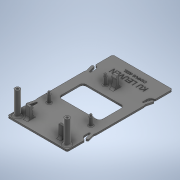
# Autodesk Inventor part: Bodemplaat_v2
Saved by Autodesk Inventor 2022 (Build 260153000, 153)
## iProperties
Created: 2022-02-17
Part Number: Bodemplaat_v2
Material: ABS Plastic
Document SubType Name: Modeling
Designer: woutr
Density: 1.06 g/cm^3
Appearance: Smooth - Black
Author: woutr
Autodesk Inventor part; units mm, degrees
note: some values were not read from the file. Chosen so that the rebuilt part matches the saved one: direction of "Emboss2".
sketch "Sketch1" plane through (0, 0, 0) normal (0, 1, 0) x (-1, 0, 0)
  line L0 (0, 0) -> (72, 0)
  line L1 (72, 0) -> (72, -127)
  line L2 (72, -127) -> (0, -127)
  line L3 (0, -127) -> (0, 0)
  line L4 (57, -50) -> (15, -50)
  line L5 (11, -54) -> (11, -76)
  line L6 (15, -80) -> (57, -80)
  line L7 (61, -76) -> (61, -54)
  arc A0 (11, -76) -> (15, -80) centre (15, -76) ccw
  arc A1 (57, -80) -> (61, -76) centre (57, -76) ccw
  arc A2 (15, -50) -> (11, -54) centre (15, -54) ccw
  arc A3 (61, -54) -> (57, -50) centre (57, -54) ccw
  point P0 (61, -50)
  point P1 (11, -80)
  point P2 (11, -50)
  point P3 (36, -50)
  point P4 (36, 0)
  dimension "d0" = 72
  dimension "d1" = 127
  dimension "d124" = 50
  dimension "d125" = 30
  dimension "d126" = 50
  dimension "d127" = 4
  constraints: 16 end point, 8 point on circle, 8 tangent, 6 point on line, 4 centre point, 4 parallel, 3 equal radius, 2 horizontal, 2 midpoint, 2 perpendicular, 1 vertical alignment
  measures "d0" distance of L1.end L2.end
  measures "d1" distance of L0.end L1.end
  measures "d124" distance between parallel lines of L0 L4
  measures "d125" distance of point (11, -50) point (11, -80)
  measures "d126" distance of point (61, -50) point (11, -50)
  measures "d127" radius of A0
extrude "Extrusion1" add sketch "Sketch1" along normal blind 2
sketch "Sketch2" plane through (0, 2, 0) normal (0, 1, 0) x (1, 0, 0)
  circle A0 centre (-60.5, 38.7) radius 2
  circle A1 centre (-11.5, 40) radius 2
  circle A2 centre (-45.2, 91.15) radius 2
  line L0 (-71, 11) -> (-1, 11) construction
  line L1 (-1, 11) -> (-1, 93.45) construction
  line L2 (-1, 93.45) -> (-71, 93.45) construction
  line L3 (-71, 93.45) -> (-71, 11) construction
  line L4 (-72, 0) -> (0, 0) projected
  point P0 (-36, 11)
  point P1 (-36, 0)
  dimension "d34" = 4
  dimension "d83" = 70
  dimension "d84" = 82.45
  dimension "d85" = 29
  dimension "d86" = 10.5
  dimension "d87" = 25.8
  dimension "d88" = 10.5
  dimension "d89" = 2.3
  dimension "d90" = 11
  dimension "d123" = 27.7
  constraints: 8 end point, 3 centre point, 2 equal radius, 2 horizontal, 2 midpoint, 2 perpendicular, 1 vertical alignment
  measures "d34" diameter of A1
  measures "d83" distance between parallel lines of L1 L3
  measures "d84" distance between parallel lines of L2 L0
  measures "d85" distance from line of L0 A1.centre
  measures "d86" distance from line of L1 A1.centre
  measures "d87" distance from line of L3 A2.centre
  measures "d88" distance from line of L3 A0.centre
  measures "d89" distance from line of L2 A2.centre
  measures "d90" distance between parallel lines of L4 L0
  measures "d123" distance from line of L0 A0.centre
extrude "Extrusion8" add sketch "Sketch2" along normal blind 9
fillet "Fillet3" radius 1 3 edges at (-62.5, 2, -38.7) (-13.5, 2, -40) (-47.2, 2, -91.15)
sketch "Sketch8" plane through (-60.5, 11, -38.7) normal (0, 1, 0) x (1, 0, 0)
  circle A0 centre (0, 0) radius 1.25
  circle A1 centre (49, 1.3) radius 2 projected
  circle A2 centre (49, 1.3) radius 1.25
  circle A3 centre (15.3, 52.45) radius 2 projected
  circle A4 centre (15.3, 52.45) radius 1.25
  circle A5 centre (0, 0) radius 2 projected
  point P0 (60.5, -38.7)
  dimension "d65" = 2.5
  dimension "d66" = 2.5
  dimension "d67" = 2.5
  constraints: 3 centre point, 2 coincident, 1 concentric
  measures "d65" diameter of A0
  measures "d66" diameter of A2
  measures "d67" diameter of A4
extrude "Extrusion9" add sketch "Sketch8" along normal blind 3 contours A0 | A2 | A4
fillet "Fillet4" radius 0.5 3 edges at (-61.75, 14, -38.7) (-12.75, 14, -40) (-46.45, 14, -91.15)
fillet "Fillet5" radius 2 4 edges at (0, 1, 0) (-72, 1, 0) (-72, 1, -127) (0, 1, -127)
ref_plane "Work Plane1" through (-16, 0, -2) normal (1, 0, 0) x (0, 0, -1)
sketch "Sketch10" plane through (-16, 0, -2) normal (1, 0, 0) x (0, 0, -1)
  line L0 (0, 2) -> (123, 2) projected
  line L1 (3.5, 2) -> (13.5, 2)
  arc A0 (10.7088, 3.9004) -> (13.5, 2) centre (13.5, 5) ccw
  arc A1 (3.5, 2) -> (6.5, 5) centre (3.5, 5) ccw
  line L2 (6.5, 5) -> (6.5, 15.9)
  line L3 (6.5, 15.9) -> (9, 15.9)
  line L4 (9, 15.9) -> (10.5, 13.9)
  line L5 (10.5, 13.9) -> (10.5, 12.9)
  line L6 (10.5, 12.9) -> (9, 12.9)
  arc A2 (9, 12.9) -> (10.7088, 3.9004) centre (33.5533, 12.9) ccw
  line L7 (-2, 2) -> (-2, 0) projected
  dimension "d92" = 10
  dimension "d96" = 1
  dimension "d98" = 3
  dimension "d100" = 2.5
  dimension "d102" = 1.5
  dimension "d103" = 3
  dimension "d117" = 10.9
  dimension "d121" = 5.5
  constraints: 12 end point, 6 point on circle, 4 tangent, 3 centre point, 3 point on line, 2 perpendicular, 1 equal radius, 1 parallel, 1 vertical, 1 vertical alignment
  measures "d92" distance of L1.start L1.end
  measures "d96" distance of L4.end L5.end
  measures "d98" radius of A0
  measures "d100" horizontal distance of L2.end L6.end
  measures "d102" distance of L5.end L6.end
  measures "d103" distance between parallel lines of L3 L6
  measures "d117" distance between parallel lines of L6 L1
  measures "d121" distance from line of L7 L1.start
extrude "Extrusion11" add sketch "Sketch10" along normal mid plane 5
ref_plane "Work Plane2" through (-36, 0, -2) normal (1, 0, 0) x (0, 0, -1)
mirror "Mirror1" about plane through (-36, 0, -2) normal (1, 0, 0) of "Extrusion11"
sketch "Sketch11" plane through (-36, 0, -2) normal (1, 0, 0) x (0, 0, -1)
  line L0 (0, 2) -> (123, 2) projected
  line L1 (86.95, 2) -> (96.95, 2)
  arc A0 (93.95, 5) -> (96.95, 2) centre (96.95, 5) ccw
  line L2 (93.95, 5) -> (93.95, 15.9)
  line L3 (93.95, 15.9) -> (91.45, 15.9)
  line L4 (91.45, 15.9) -> (89.95, 13.9)
  line L5 (89.95, 13.9) -> (89.95, 12.9)
  line L6 (89.95, 12.9) -> (91.45, 12.9)
  arc A1 (86.95, 2) -> (89.7412, 3.9004) centre (86.95, 5) ccw
  arc A2 (89.7412, 3.9004) -> (91.45, 12.9) centre (66.8967, 12.9) ccw
  line L7 (-2, 2) -> (-2, 0) projected
  point P0 (9, 12.9)
  dimension "d107" = 10
  dimension "d109" = 2.5
  dimension "d112" = 3
  dimension "d113" = 3
  dimension "d118" = 1
  dimension "d119" = 1.5
  dimension "d120" = 10.9
  dimension "d122" = 82.45
  constraints: 12 end point, 6 point on circle, 4 tangent, 3 centre point, 3 point on line, 2 perpendicular, 1 equal radius, 1 parallel, 1 vertical, 1 vertical alignment
  measures "d107" distance of L1.start L1.end
  measures "d109" distance of L2.end L3.end
  measures "d112" radius of A0
  measures "d113" distance between parallel lines of L3 L6
  measures "d118" distance of L4.end L5.end
  measures "d119" distance of L5.end L6.end
  measures "d120" distance between parallel lines of L1 L6
  measures "d122" distance of L6.end point (9, 12.9)
extrude "Extrusion12" add sketch "Sketch11" along normal mid plane 5
sketch "Sketch12" plane through (0, 2, 0) normal (0, 1, 0) x (1, 0, 0)
  circle A0 centre (-66, 6) radius 3
  line L0 (-72, 125) -> (-72, 2) projected
  line L1 (-70, 0) -> (-2, 0) projected
  circle A1 centre (-6, 6) radius 3
  line L2 (0, 2) -> (0, 125) projected
  point P0 (0, 0)
  dimension "d128" = 6
  dimension "d129" = 6
  dimension "d130" = 6
  dimension "d131" = 6
  dimension "d132" = 6
  constraints: 2 centre point, 1 equal radius
  measures "d128" diameter of A0
  measures "d129" distance from line of L0 A0.centre
  measures "d130" distance from line of L1 A0.centre
  measures "d131" distance from line of L2 A1.centre
  measures "d132" distance from line of L1 A1.centre
extrude "Extrusion13" add sketch "Sketch12" along normal blind 28
fillet "Fillet6" radius 2 2 edges at (-9, 2, -6) (-69, 2, -6)
sketch "Sketch13" plane through (-6, 30, -6) normal (0, 1, 0) x (1, 0, 0)
  circle A0 centre (0, 0) radius 3 projected
  circle A1 centre (0, 0) radius 1.25
  circle A2 centre (-60, 0) radius 3 projected
  circle A3 centre (-60, 0) radius 1.25
  point P0 (6, -6)
  dimension "d136" = 2.5
  dimension "d137" = 2.5
  constraints: 2 centre point, 2 coincident
  measures "d136" diameter of A1
  measures "d137" diameter of A3
extrude "Extrusion14" cut sketch "Sketch13" against normal blind 10 contours A1 | A3
sketch "Sketch16" plane through (0, 2, 0) normal (0, 1, 0) x (1, 0, 0)
  line L0 (-14.5113, 107.1159) -> (-57.4887, 107.1159) construction
  line L1 (-57.4887, 107.1159) -> (-57.4887, 122) construction
  line L2 (-57.4887, 122) -> (-14.5113, 122) construction
  line L3 (-14.5113, 122) -> (-14.5113, 107.1159) construction
  line L4 (-2, 127) -> (-70, 127) projected
  line L5 (-19.6921, 113.2159) -> (-18.6392, 113.2159)
  line L6 (-18.6392, 113.2159) -> (-16.4098, 110.3785)
  line L7 (-16.4098, 110.3785) -> (-16.0539, 110.7789)
  line L8 (-16.0539, 110.7789) -> (-16.0539, 113.2159)
  line L9 (-16.0539, 113.2159) -> (-15.2432, 113.2159)
  line L10 (-15.2432, 113.2159) -> (-15.2432, 107.1159)
  line L11 (-15.2432, 107.1159) -> (-16.0539, 107.1159)
  line L12 (-16.0539, 107.1159) -> (-16.0539, 109.9187)
  line L13 (-16.0539, 109.9187) -> (-18.5552, 107.1159)
  line L14 (-18.5552, 107.1159) -> (-19.5438, 107.1159)
  line L15 (-19.5438, 107.1159) -> (-17.0178, 109.8396)
  line L16 (-17.0178, 109.8396) -> (-19.6921, 113.2159)
  spline S0 degree 2 poles (-22.3071, 113.3444) (-21.7683, 113.3444) (-20.9675, 113.0626) (-20.6857, 112.7809) knots 0 0 0 1 2 2 2
  spline S1 degree 2 poles (-20.6857, 112.7809) (-20.3644, 112.4645) (-20.1024, 111.5747) (-20.1024, 110.9222) knots 0 0 0 1 2 2 2
  line L17 (-20.1024, 110.9222) -> (-20.1024, 107.1159)
  line L18 (-20.1024, 107.1159) -> (-20.9131, 107.1159)
  line L19 (-20.9131, 107.1159) -> (-20.9131, 110.9222)
  spline S2 degree 2 poles (-20.9131, 110.9222) (-20.9131, 111.3473) (-21.0219, 111.9208) (-21.1751, 112.1531) knots 0 0 0 1 2 2 2
  spline S3 degree 2 poles (-21.1751, 112.1531) (-21.3382, 112.4003) (-21.9018, 112.6524) (-22.3071, 112.6524) knots 0 0 0 1 2 2 2
  spline S4 degree 2 poles (-22.3071, 112.6524) (-22.6878, 112.6524) (-23.281, 112.4003) (-23.4441, 112.1531) knots 0 0 0 1 2 2 2
  spline S5 degree 2 poles (-23.4441, 112.1531) (-23.5973, 111.9208) (-23.7061, 111.3523) (-23.7061, 110.942) knots 0 0 0 1 2 2 2
  line L20 (-23.7061, 110.942) -> (-23.7061, 107.1159)
  line L21 (-23.7061, 107.1159) -> (-24.5168, 107.1159)
  line L22 (-24.5168, 107.1159) -> (-24.5168, 110.9222)
  spline S6 degree 2 poles (-24.5168, 110.9222) (-24.5168, 111.5599) (-24.2597, 112.4695) (-23.9335, 112.7809) knots 0 0 0 1 2 2 2
  spline S7 degree 2 poles (-23.9335, 112.7809) (-23.6418, 113.0676) (-22.8707, 113.3444) (-22.3071, 113.3444) knots 0 0 0 1 2 2 2
  line L23 (-31.8328, 113.2159) -> (-28.2984, 113.2159)
  line L24 (-28.2984, 113.2159) -> (-28.2984, 107.1159)
  line L25 (-28.2984, 107.1159) -> (-29.1091, 107.1159)
  line L26 (-29.1091, 107.1159) -> (-29.1091, 112.4942)
  line L27 (-29.1091, 112.4942) -> (-31.8328, 112.4942)
  line L28 (-31.8328, 112.4942) -> (-31.8328, 113.2159)
  line L29 (-32.4705, 113.2159) -> (-32.4705, 107.1159)
  line L30 (-32.4705, 107.1159) -> (-36.2867, 107.1159)
  line L31 (-36.2867, 107.1159) -> (-36.2867, 107.8376)
  line L32 (-36.2867, 107.8376) -> (-33.2812, 107.8376)
  line L33 (-33.2812, 107.8376) -> (-33.2812, 109.5084)
  line L34 (-33.2812, 109.5084) -> (-36.084, 109.5084)
  line L35 (-36.084, 109.5084) -> (-36.084, 110.2302)
  line L36 (-36.084, 110.2302) -> (-33.2812, 110.2302)
  line L37 (-33.2812, 110.2302) -> (-33.2812, 112.4942)
  line L38 (-33.2812, 112.4942) -> (-36.2867, 112.4942)
  line L39 (-36.2867, 112.4942) -> (-36.2867, 113.2159)
  line L40 (-36.2867, 113.2159) -> (-32.4705, 113.2159)
  spline S8 degree 2 poles (-39.3071, 113.3444) (-38.7682, 113.3444) (-37.9674, 113.0626) (-37.6857, 112.7809) knots 0 0 0 1 2 2 2
  spline S9 degree 2 poles (-37.6857, 112.7809) (-37.3643, 112.4645) (-37.1024, 111.5747) (-37.1024, 110.9222) knots 0 0 0 1 2 2 2
  line L41 (-37.1024, 110.9222) -> (-37.1024, 107.1159)
  line L42 (-37.1024, 107.1159) -> (-37.913, 107.1159)
  line L43 (-37.913, 107.1159) -> (-37.913, 110.9222)
  spline S10 degree 2 poles (-37.913, 110.9222) (-37.913, 111.3473) (-38.0218, 111.9208) (-38.175, 112.1531) knots 0 0 0 1 2 2 2
  spline S11 degree 2 poles (-38.175, 112.1531) (-38.3382, 112.4003) (-38.9017, 112.6524) (-39.3071, 112.6524) knots 0 0 0 1 2 2 2
  spline S12 degree 2 poles (-39.3071, 112.6524) (-39.6877, 112.6524) (-40.2809, 112.4003) (-40.444, 112.1531) knots 0 0 0 1 2 2 2
  spline S13 degree 2 poles (-40.444, 112.1531) (-40.5972, 111.9208) (-40.706, 111.3523) (-40.706, 110.942) knots 0 0 0 1 2 2 2
  line L44 (-40.706, 110.942) -> (-40.706, 107.1159)
  line L45 (-40.706, 107.1159) -> (-41.5167, 107.1159)
  line L46 (-41.5167, 107.1159) -> (-41.5167, 110.9222)
  spline S14 degree 2 poles (-41.5167, 110.9222) (-41.5167, 111.5599) (-41.2596, 112.4695) (-40.9334, 112.7809) knots 0 0 0 1 2 2 2
  spline S15 degree 2 poles (-40.9334, 112.7809) (-40.6417, 113.0676) (-39.8706, 113.3444) (-39.3071, 113.3444) knots 0 0 0 1 2 2 2
  line L47 (-47.1026, 107.1159) -> (-45.0017, 113.2159)
  line L48 (-45.0017, 113.2159) -> (-44.1267, 113.2159)
  line L49 (-44.1267, 113.2159) -> (-42.0259, 107.1159)
  line L50 (-42.0259, 107.1159) -> (-42.8959, 107.1159)
  line L51 (-42.8959, 107.1159) -> (-44.5865, 112.1827)
  line L52 (-44.5865, 112.1827) -> (-46.2771, 107.1159)
  line L53 (-46.2771, 107.1159) -> (-47.1026, 107.1159)
  line L54 (-47.6859, 113.2159) -> (-47.6859, 107.1159)
  line L55 (-47.6859, 107.1159) -> (-51.5021, 107.1159)
  line L56 (-51.5021, 107.1159) -> (-51.5021, 107.8376)
  line L57 (-51.5021, 107.8376) -> (-48.4966, 107.8376)
  line L58 (-48.4966, 107.8376) -> (-48.4966, 109.5084)
  line L59 (-48.4966, 109.5084) -> (-51.2994, 109.5084)
  line L60 (-51.2994, 109.5084) -> (-51.2994, 110.2302)
  line L61 (-51.2994, 110.2302) -> (-48.4966, 110.2302)
  line L62 (-48.4966, 110.2302) -> (-48.4966, 112.4942)
  line L63 (-48.4966, 112.4942) -> (-51.5021, 112.4942)
  line L64 (-51.5021, 112.4942) -> (-51.5021, 113.2159)
  line L65 (-51.5021, 113.2159) -> (-47.6859, 113.2159)
  line L66 (-56.7568, 113.2159) -> (-55.8472, 113.2159)
  line L67 (-55.8472, 113.2159) -> (-53.1482, 107.9562)
  line L68 (-53.1482, 107.9562) -> (-53.1482, 113.2159)
  line L69 (-53.1482, 113.2159) -> (-52.3919, 113.2159)
  line L70 (-52.3919, 113.2159) -> (-52.3919, 107.1159)
  line L71 (-52.3919, 107.1159) -> (-53.5437, 107.1159)
  line L72 (-53.5437, 107.1159) -> (-56.0005, 111.9455)
  line L73 (-56.0005, 111.9455) -> (-56.0005, 107.1159)
  line L74 (-56.0005, 107.1159) -> (-56.7568, 107.1159)
  line L75 (-56.7568, 107.1159) -> (-56.7568, 113.2159)
  spline S16 degree 2 poles (-24.223, 119.4664) (-23.9266, 119.4664) (-23.4251, 119.2664) (-23.2424, 119.0663) knots 0 0 0 1 2 2 2
  spline S17 degree 2 poles (-23.2424, 119.0663) (-23.0596, 118.8687) (-22.8595, 118.2759) (-22.8595, 117.8906) knots 0 0 0 1 2 2 2
  spline S18 degree 2 poles (-22.8595, 117.8906) (-22.8595, 117.5077) (-23.0546, 116.9396) (-23.2399, 116.7297) knots 0 0 0 1 2 2 2
  spline S19 degree 2 poles (-23.2399, 116.7297) (-23.4227, 116.5246) (-23.9216, 116.3098) (-24.2304, 116.3098) knots 0 0 0 1 2 2 2
  spline S20 degree 2 poles (-24.2304, 116.3098) (-24.3835, 116.3098) (-24.6527, 116.3542) (-24.7664, 116.3888) knots 0 0 0 1 2 2 2
  spline S21 degree 2 poles (-24.7664, 116.3888) (-24.8652, 116.4209) (-25.0702, 116.5123) (-25.1714, 116.5666) knots 0 0 0 1 2 2 2
  line L76 (-25.1714, 116.5666) -> (-25.1714, 117.0557)
  line L77 (-25.1714, 117.0557) -> (-25.1393, 117.0557)
  spline S22 degree 2 poles (-25.1393, 117.0557) (-25.085, 117.0063) (-24.917, 116.868) (-24.796, 116.8013) knots 0 0 0 1 2 2 2
  spline S23 degree 2 poles (-24.796, 116.8013) (-24.6799, 116.7371) (-24.4057, 116.6556) (-24.2279, 116.6556) knots 0 0 0 1 2 2 2
  spline S24 degree 2 poles (-24.2279, 116.6556) (-24.0328, 116.6556) (-23.6845, 116.8161) (-23.5536, 116.9692) knots 0 0 0 1 2 2 2
  spline S25 degree 2 poles (-23.5536, 116.9692) (-23.4251, 117.1249) (-23.2819, 117.5966) (-23.2819, 117.8906) knots 0 0 0 1 2 2 2
  spline S26 degree 2 poles (-23.2819, 117.8906) (-23.2819, 118.2043) (-23.4326, 118.6563) (-23.5635, 118.8119) knots 0 0 0 1 2 2 2
  spline S27 degree 2 poles (-23.5635, 118.8119) (-23.6919, 118.9625) (-24.0352, 119.1157) (-24.2279, 119.1157) knots 0 0 0 1 2 2 2
  spline S28 degree 2 poles (-24.2279, 119.1157) (-24.4033, 119.1157) (-24.7021, 119.0292) (-24.8182, 118.965) knots 0 0 0 1 2 2 2
  spline S29 degree 2 poles (-24.8182, 118.965) (-24.9294, 118.9008) (-25.0949, 118.7674) (-25.1418, 118.7205) knots 0 0 0 1 2 2 2
  line L78 (-25.1418, 118.7205) -> (-25.1714, 118.7205)
  line L79 (-25.1714, 118.7205) -> (-25.1714, 119.2046)
  spline S30 degree 2 poles (-25.1714, 119.2046) (-25.0702, 119.2515) (-24.8923, 119.338) (-24.7664, 119.3775) knots 0 0 0 1 2 2 2
  spline S31 degree 2 poles (-24.7664, 119.3775) (-24.633, 119.422) (-24.4057, 119.4664) (-24.223, 119.4664) knots 0 0 0 1 2 2 2
  line L80 (-25.2208, 119.4121) -> (-26.2484, 116.3641)
  line L81 (-26.2484, 116.3641) -> (-26.7473, 116.3641)
  line L82 (-26.7473, 116.3641) -> (-27.7748, 119.4121)
  line L83 (-27.7748, 119.4121) -> (-27.3475, 119.4121)
  line L84 (-27.3475, 119.4121) -> (-27.0709, 118.5599)
  line L85 (-27.0709, 118.5599) -> (-25.9075, 118.5599)
  line L86 (-25.9075, 118.5599) -> (-25.6309, 119.4121)
  line L87 (-25.6309, 119.4121) -> (-25.2208, 119.4121)
  line L88 (-26.9597, 118.2141) -> (-26.488, 116.7791)
  line L89 (-26.488, 116.7791) -> (-26.0187, 118.2141)
  line L90 (-26.0187, 118.2141) -> (-26.9597, 118.2141)
  line L91 (-30.6771, 119.4121) -> (-30.272, 119.4121)
  line L92 (-30.272, 119.4121) -> (-30.272, 116.7865)
  line L93 (-30.272, 116.7865) -> (-29.4767, 118.5723)
  line L94 (-29.4767, 118.5723) -> (-29.2297, 118.5723)
  line L95 (-29.2297, 118.5723) -> (-28.4418, 116.7865)
  line L96 (-28.4418, 116.7865) -> (-28.4418, 119.4121)
  line L97 (-28.4418, 119.4121) -> (-28.0638, 119.4121)
  line L98 (-28.0638, 119.4121) -> (-28.0638, 116.3641)
  line L99 (-28.0638, 116.3641) -> (-28.6171, 116.3641)
  line L100 (-28.6171, 116.3641) -> (-29.3779, 118.061)
  line L101 (-29.3779, 118.061) -> (-30.114, 116.3641)
  line L102 (-30.114, 116.3641) -> (-30.6771, 116.3641)
  line L103 (-30.6771, 116.3641) -> (-30.6771, 119.4121)
  spline S32 degree 2 poles (-33.2212, 117.2829) (-33.2212, 117.4805) (-33.0804, 117.8362) (-32.9545, 117.9597) knots 0 0 0 1 2 2 2
  spline S33 degree 2 poles (-32.9545, 117.9597) (-32.7964, 118.1153) (-32.3691, 118.2759) (-32.043, 118.2759) knots 0 0 0 1 2 2 2
  line L104 (-32.043, 118.2759) -> (-31.6997, 118.2759)
  line L105 (-31.6997, 118.2759) -> (-31.6997, 119.4121)
  line L106 (-31.6997, 119.4121) -> (-31.2946, 119.4121)
  line L107 (-31.2946, 119.4121) -> (-31.2946, 116.3641)
  line L108 (-31.2946, 116.3641) -> (-32.0603, 116.3641)
  spline S34 degree 2 poles (-32.0603, 116.3641) (-32.332, 116.3641) (-32.7124, 116.453) (-32.8581, 116.5543) knots 0 0 0 1 2 2 2
  spline S35 degree 2 poles (-32.8581, 116.5543) (-33.0286, 116.6704) (-33.2212, 117.0285) (-33.2212, 117.2829) knots 0 0 0 1 2 2 2
  spline S36 degree 2 poles (-32.7989, 117.2953) (-32.7989, 117.1372) (-32.6902, 116.905) (-32.579, 116.8309) knots 0 0 0 1 2 2 2
  spline S37 degree 2 poles (-32.579, 116.8309) (-32.4827, 116.7667) (-32.2258, 116.7148) (-32.0356, 116.7148) knots 0 0 0 1 2 2 2
  line L109 (-32.0356, 116.7148) -> (-31.6997, 116.7148)
  line L110 (-31.6997, 116.7148) -> (-31.6997, 117.9301)
  line L111 (-31.6997, 117.9301) -> (-31.9763, 117.9301)
  spline S38 degree 2 poles (-31.9763, 117.9301) (-32.2233, 117.9301) (-32.5272, 117.851) (-32.626, 117.7473) knots 0 0 0 1 2 2 2
  spline S39 degree 2 poles (-32.626, 117.7473) (-32.7173, 117.6559) (-32.7989, 117.441) (-32.7989, 117.2953) knots 0 0 0 1 2 2 2
  spline S40 degree 2 poles (-34.6711, 119.4763) (-34.4019, 119.4763) (-34.0018, 119.3355) (-33.861, 119.1947) knots 0 0 0 1 2 2 2
  spline S41 degree 2 poles (-33.861, 119.1947) (-33.7004, 119.0367) (-33.5695, 118.592) (-33.5695, 118.266) knots 0 0 0 1 2 2 2
  line L112 (-33.5695, 118.266) -> (-33.5695, 116.3641)
  line L113 (-33.5695, 116.3641) -> (-33.9746, 116.3641)
  line L114 (-33.9746, 116.3641) -> (-33.9746, 118.266)
  spline S42 degree 2 poles (-33.9746, 118.266) (-33.9746, 118.4784) (-34.0289, 118.7649) (-34.1055, 118.881) knots 0 0 0 1 2 2 2
  spline S43 degree 2 poles (-34.1055, 118.881) (-34.187, 119.0045) (-34.4686, 119.1305) (-34.6711, 119.1305) knots 0 0 0 1 2 2 2
  spline S44 degree 2 poles (-34.6711, 119.1305) (-34.8613, 119.1305) (-35.1577, 119.0045) (-35.2392, 118.881) knots 0 0 0 1 2 2 2
  spline S45 degree 2 poles (-35.2392, 118.881) (-35.3158, 118.7649) (-35.3701, 118.4809) (-35.3701, 118.2759) knots 0 0 0 1 2 2 2
  line L115 (-35.3701, 118.2759) -> (-35.3701, 116.3641)
  line L116 (-35.3701, 116.3641) -> (-35.7752, 116.3641)
  line L117 (-35.7752, 116.3641) -> (-35.7752, 118.266)
  spline S46 degree 2 poles (-35.7752, 118.266) (-35.7752, 118.5846) (-35.6468, 119.0391) (-35.4838, 119.1947) knots 0 0 0 1 2 2 2
  spline S47 degree 2 poles (-35.4838, 119.1947) (-35.338, 119.338) (-34.9527, 119.4763) (-34.6711, 119.4763) knots 0 0 0 1 2 2 2
  spline S48 degree 2 poles (-37.2054, 119.4664) (-36.8744, 119.4664) (-36.41, 119.3281) (-36.205, 119.2293) knots 0 0 0 1 2 2 2
  line L118 (-36.205, 119.2293) -> (-36.205, 118.7205)
  line L119 (-36.205, 118.7205) -> (-36.2347, 118.7205)
  spline S49 degree 2 poles (-36.2347, 118.7205) (-36.4347, 118.9082) (-36.9411, 119.1157) (-37.1757, 119.1157) knots 0 0 0 1 2 2 2
  spline S50 degree 2 poles (-37.1757, 119.1157) (-37.5116, 119.1157) (-37.855, 118.8366) (-37.855, 118.6069) knots 0 0 0 1 2 2 2
  spline S51 degree 2 poles (-37.855, 118.6069) (-37.855, 118.4241) (-37.6747, 118.1968) (-37.4795, 118.14) knots 0 0 0 1 2 2 2
  spline S52 degree 2 poles (-37.4795, 118.14) (-37.3387, 118.1005) (-37.1041, 118.0462) (-36.9287, 118.0017) knots 0 0 0 1 2 2 2
  spline S53 degree 2 poles (-36.9287, 118.0017) (-36.7706, 117.9597) (-36.5212, 117.8338) (-36.4248, 117.7325) knots 0 0 0 1 2 2 2
  spline S54 degree 2 poles (-36.4248, 117.7325) (-36.331, 117.6312) (-36.2272, 117.3595) (-36.2272, 117.1817) knots 0 0 0 1 2 2 2
  spline S55 degree 2 poles (-36.2272, 117.1817) (-36.2272, 116.8112) (-36.8052, 116.3098) (-37.2523, 116.3098) knots 0 0 0 1 2 2 2
  spline S56 degree 2 poles (-37.2523, 116.3098) (-37.5092, 116.3098) (-37.9637, 116.411) (-38.1588, 116.5074) knots 0 0 0 1 2 2 2
  line L120 (-38.1588, 116.5074) -> (-38.1588, 116.9915)
  line L121 (-38.1588, 116.9915) -> (-38.1292, 116.9915)
  spline S57 degree 2 poles (-38.1292, 116.9915) (-37.9834, 116.8581) (-37.5289, 116.6605) (-37.2795, 116.6605) knots 0 0 0 1 2 2 2
  spline S58 degree 2 poles (-37.2795, 116.6605) (-36.9979, 116.6605) (-36.6496, 116.9248) (-36.6496, 117.1397) knots 0 0 0 1 2 2 2
  spline S59 degree 2 poles (-36.6496, 117.1397) (-36.6496, 117.3323) (-36.8546, 117.5621) (-37.0473, 117.6139) knots 0 0 0 1 2 2 2
  spline S60 degree 2 poles (-37.0473, 117.6139) (-37.1757, 117.6485) (-37.5487, 117.7374) (-37.6722, 117.7745) knots 0 0 0 1 2 2 2
  spline S61 degree 2 poles (-37.6722, 117.7745) (-37.9859, 117.8708) (-38.2774, 118.2586) (-38.2774, 118.5426) knots 0 0 0 1 2 2 2
  spline S62 degree 2 poles (-38.2774, 118.5426) (-38.2774, 118.723) (-38.1316, 119.0688) (-38.0007, 119.1898) knots 0 0 0 1 2 2 2
  spline S63 degree 2 poles (-38.0007, 119.1898) (-37.855, 119.3232) (-37.4845, 119.4664) (-37.2054, 119.4664) knots 0 0 0 1 2 2 2
  spline S64 degree 2 poles (-41.276, 119.4714) (-40.9524, 119.4714) (-40.4164, 119.2738) (-40.2237, 119.0737) knots 0 0 0 1 2 2 2
  spline S65 degree 2 poles (-40.2237, 119.0737) (-40.0311, 118.8712) (-39.8261, 118.2734) (-39.8261, 117.8856) knots 0 0 0 1 2 2 2
  spline S66 degree 2 poles (-39.8261, 117.8856) (-39.8261, 117.5176) (-40.0335, 116.9347) (-40.2262, 116.7272) knots 0 0 0 1 2 2 2
  spline S67 degree 2 poles (-40.2262, 116.7272) (-40.4114, 116.5271) (-40.9549, 116.3098) (-41.2784, 116.3098) knots 0 0 0 1 2 2 2
  spline S68 degree 2 poles (-41.2784, 116.3098) (-41.434, 116.3098) (-41.7156, 116.3542) (-41.8441, 116.3937) knots 0 0 0 1 2 2 2
  spline S69 degree 2 poles (-41.8441, 116.3937) (-41.9478, 116.4234) (-42.1997, 116.5321) (-42.2763, 116.5716) knots 0 0 0 1 2 2 2
  line L122 (-42.2763, 116.5716) -> (-42.2763, 117.0606)
  line L123 (-42.2763, 117.0606) -> (-42.2417, 117.0606)
  spline S70 degree 2 poles (-42.2417, 117.0606) (-42.1652, 116.9939) (-42.0046, 116.8729) (-41.8564, 116.8038) knots 0 0 0 1 2 2 2
  spline S71 degree 2 poles (-41.8564, 116.8038) (-41.7329, 116.742) (-41.4143, 116.6605) (-41.2315, 116.6605) knots 0 0 0 1 2 2 2
  spline S72 degree 2 poles (-41.2315, 116.6605) (-40.7918, 116.6605) (-40.2484, 117.3225) (-40.2484, 117.8733) knots 0 0 0 1 2 2 2
  spline S73 degree 2 poles (-40.2484, 117.8733) (-40.2484, 118.1796) (-40.3917, 118.639) (-40.5275, 118.7971) knots 0 0 0 1 2 2 2
  spline S74 degree 2 poles (-40.5275, 118.7971) (-40.6585, 118.9551) (-41.029, 119.1206) (-41.2611, 119.1206) knots 0 0 0 1 2 2 2
  spline S75 degree 2 poles (-41.2611, 119.1206) (-41.4316, 119.1206) (-41.7724, 119.0712) (-41.8885, 119.0218) knots 0 0 0 1 2 2 2
  line L124 (-41.8885, 119.0218) -> (-41.8885, 118.2339)
  line L125 (-41.8885, 118.2339) -> (-41.1821, 118.2339)
  line L126 (-41.1821, 118.2339) -> (-41.1821, 117.8782)
  line L127 (-41.1821, 117.8782) -> (-42.2887, 117.8782)
  line L128 (-42.2887, 117.8782) -> (-42.2887, 119.2096)
  spline S76 degree 2 poles (-42.2887, 119.2096) (-42.2121, 119.2441) (-41.9503, 119.3503) (-41.8391, 119.3825) knots 0 0 0 1 2 2 2
  spline S77 degree 2 poles (-41.8391, 119.3825) (-41.6884, 119.4269) (-41.4464, 119.4714) (-41.276, 119.4714) knots 0 0 0 1 2 2 2
  line L129 (-42.7975, 119.4121) -> (-42.7975, 116.3641)
  line L130 (-42.7975, 116.3641) -> (-44.7043, 116.3641)
  line L131 (-44.7043, 116.3641) -> (-44.7043, 116.7247)
  line L132 (-44.7043, 116.7247) -> (-43.2026, 116.7247)
  line L133 (-43.2026, 116.7247) -> (-43.2026, 117.5596)
  line L134 (-43.2026, 117.5596) -> (-44.6031, 117.5596)
  line L135 (-44.6031, 117.5596) -> (-44.6031, 117.9202)
  line L136 (-44.6031, 117.9202) -> (-43.2026, 117.9202)
  line L137 (-43.2026, 117.9202) -> (-43.2026, 119.0515)
  line L138 (-43.2026, 119.0515) -> (-44.7043, 119.0515)
  line L139 (-44.7043, 119.0515) -> (-44.7043, 119.4121)
  line L140 (-44.7043, 119.4121) -> (-42.7975, 119.4121)
  line L141 (-45.1489, 119.4121) -> (-45.1489, 116.3641)
  line L142 (-45.1489, 116.3641) -> (-47.0558, 116.3641)
  line L143 (-47.0558, 116.3641) -> (-47.0558, 116.7247)
  line L144 (-47.0558, 116.7247) -> (-45.554, 116.7247)
  line L145 (-45.554, 116.7247) -> (-45.554, 117.5596)
  line L146 (-45.554, 117.5596) -> (-46.9545, 117.5596)
  line L147 (-46.9545, 117.5596) -> (-46.9545, 117.9202)
  line L148 (-46.9545, 117.9202) -> (-45.554, 117.9202)
  line L149 (-45.554, 117.9202) -> (-45.554, 119.0515)
  line L150 (-45.554, 119.0515) -> (-47.0558, 119.0515)
  line L151 (-47.0558, 119.0515) -> (-47.0558, 119.4121)
  line L152 (-47.0558, 119.4121) -> (-45.1489, 119.4121)
  line L153 (-49.2665, 119.4121) -> (-47.5004, 119.4121)
  line L154 (-47.5004, 119.4121) -> (-47.5004, 116.3641)
  line L155 (-47.5004, 116.3641) -> (-47.9055, 116.3641)
  line L156 (-47.9055, 116.3641) -> (-47.9055, 119.0515)
  line L157 (-47.9055, 119.0515) -> (-49.2665, 119.0515)
  line L158 (-49.2665, 119.0515) -> (-49.2665, 119.4121)
  point P0 (0, 0)
  point P1 (-36, 122)
  point P2 (-36, 127)
  dimension "d162" = 5
  constraints: 2 midpoint, 1 vertical alignment, 2 other
  measures "d162" distance from line of L4 point (-36, 122)
emboss "Emboss2" sketch "Sketch16" operation cut depth 1 direction (0, -1, 0)
sketch "Sketch19" plane through (0, 2, 0) normal (0, 1, 0) x (1, 0, 0)
  line L0 (0, 2) -> (0, 125) projected
  line L1 (0, 35) -> (-5, 35)
  line L2 (-70, 0) -> (-2, 0) projected
  line L3 (-2, 127) -> (-70, 127) projected
  line L4 (-5, 35) -> (-5, 20)
  line L5 (-5, 20) -> (0, 20)
  point P0 (0, 0)
  point P1 (-2.5, 35)
  dimension "d182" = 5
  dimension "d185" = 20
  dimension "d188" = 15
  constraints: 6 end point, 2 perpendicular, 2 point on line, 1 midpoint, 1 vertical
  measures "d182" distance of L1.start L1.end
  measures "d185" distance from line of L2 L5.end
  measures "d188" vertical distance of L5.end point (-2.5, 35)
extrude "Extrusion15" cut sketch "Sketch19" against normal through all
sketch "Sketch20" plane through (0, 2, 0) normal (0, 1, 0) x (1, 0, 0)
  line L0 (-5, 20) -> (-5, 35) projected
  line L1 (-5, 35) -> (0, 35) projected
  line L2 (1.4489, 24.8882) -> (-0.4549, 31.9933)
  arc A0 (-1.4489, 24.1118) -> (1.4489, 24.8882) centre (0, 24.5) ccw
  line L3 (-1.4489, 24.1118) -> (-3.3527, 31.2169)
  arc A1 (-3.3527, 31.2169) -> (-5, 31) centre (-4.1621, 31) ccw
  arc A2 (-0.2722, 33.8362) -> (-0.4549, 31.9933) centre (2.0798, 32.6725) ccw
  line L4 (0, 35) -> (0, 125) projected
  arc A3 (-0.2722, 33.8362) -> (0, 35) centre (-2.6241, 35) ccw
  line L5 (0, 35) -> (0, 20) projected
  line L6 (-5, 23) -> (0, 23) construction
  line L7 (0, 20) -> (-5, 20) projected
  line L8 (1.5, 35) -> (1.5, 20) construction
  line L9 (0, 2) -> (0, 20) projected
  arc A4 (-5, 26) -> (-1.25, 21.5) centre (-0.425, 26) ccw
  arc A5 (0, 20) -> (-1.25, 21.5) centre (-1.525, 20) ccw
  point P0 (0, 0)
  point P1 (0, 92)
  dimension "d195" = 3
  dimension "d196" = 4
  dimension "d197" = 3
  dimension "d199" = 1.5
  dimension "d200" = 15
  dimension "d201" = 6
  dimension "d202" = 1.5
  constraints: 12 point on circle, 12 tangent, 8 end point, 6 centre point, 2 horizontal alignment, 2 parallel, 2 point on line, 1 equal radius, 1 horizontal, 1 vertical, 1 vertical alignment
  measures "d195" distance between parallel lines of L3 L2
  measures "d196" distance from line of L1 A1.end
  measures "d197" distance between parallel lines of L7 L6
  measures "d199" distance between parallel lines of L9 L8
  measures "d200" angle of L0 L3
  measures "d201" distance of L0.start A4.start
  measures "d202" distance from line of L7 A4.end
extrude "Extrusion16" add sketch "Sketch20" against normal up to surface (2 mm away) contours L0 A4 A5 L7 | L0 L1 A3 A2 L2 L5 A0 L3 A1 | L5 L2 A0
ref_plane "Work Plane3" through (-70, 0, -63.5) normal (0, 0, 1) x (1, 0, 0)
mirror "Mirror4" about plane through (-36, 0, -2) normal (1, 0, 0) of "Extrusion16", "Extrusion15"
mirror "Mirror5" about plane through (-70, 0, -63.5) normal (0, 0, 1) of "Extrusion15", "Extrusion16", "Mirror4"
body "Solid1"
